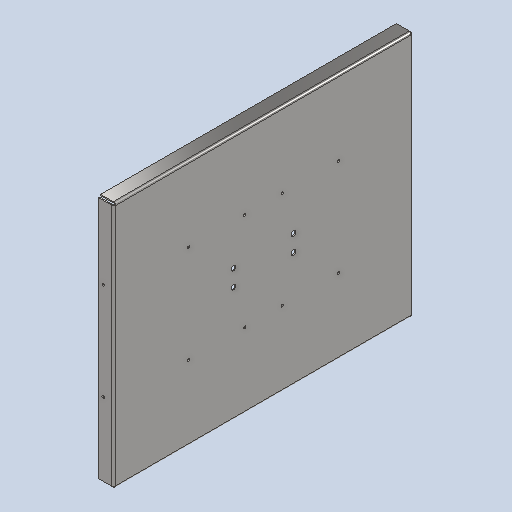
# Autodesk Inventor part: C_plate
Saved by Autodesk Inventor 2025.2 (Build 292293000, 293)
## iProperties
Created: 2025-04-08
Part Number: C_plate
Material: Stainless Steel
Document SubType Name: Sheet Metal
Designer: Caspe
Density: 8 g/cm^3
Sheet Metal Rule: Default_mm
Appearance: Semi-Polished
Flat Pattern Width: 36.4786 cm
Flat Pattern Length: 43.4786 cm
Flat Pattern Area: 1586.04 cm^2
Sheet Metal Width: 364,786 mm
Sheet Metal Length: 434,786 mm
Sheet Metal Area: 158603,718 mm^2
Mass: 1883.49 g
Surface Area: 3166.42 cm^2
Volume: 235.436 cm^3
Author: Caspe
Autodesk Inventor part; units mm, degrees
note: some values were not read from the file. Chosen so that the rebuilt part matches the saved one: corner form of "Plate2".
ref_plane "YZ Plane" through (0, 0, 0) normal (1, 0, 0) x (0, 1, 0)
ref_plane "XZ Plane" through (0, 0, 0) normal (0, 1, 0) x (-1, 0, 0)
ref_plane "XY Plane" through (0, 0, 0) normal (0, 0, 1) x (1, 0, 0)
sketch "Sketch1" plane through (0, 0, 0) normal (1, 0, 0) x (0, 1, 0)
  line L0 (165, 200) -> (-165, 200)
  line L1 (-165, 200) -> (-165, -200)
  line L2 (-165, -200) -> (165, -200)
  line L3 (165, -200) -> (165, 200)
  line L4 (165, 200) -> (-165, -200) construction
  line L5 (-165, 200) -> (165, -200) construction
  point P0 (0, 0)
  dimension "d0" = 330
  dimension "d1" = 400
  measures "d0" distance of L2.end L1.end
  measures "d1" distance of L1.end L0.end
extrude "Plate1" add sketch "Sketch1" along normal blind 1.5
sketch "Sketch2" plane through (1.5, 165, 198.5) normal (0, 0, 1) x (1, 0, 0)
  line L0 (0, -330) -> (0, 0)
  line L1 (0, 0) -> (-20, 0)
  line L2 (-20, 0) -> (-20, -330)
  line L3 (-20, -330) -> (0, -330)
  constraints: 6 end point, 1 horizontal, 1 perpendicular, 1 vertical
edge flange "Flange1" height 20 angle 90 thickness 1.5 bend radius 1.5 thickness toward (0, 0, 1) relief tear relief width 1.5 relief depth 0.75 corner gap 1.5 corner form 2 edges at (0, 0, 200) (0, 165, 0) (0, 0, -200) (0, -165, 0) wall of the first edge with corners at (1.5, -165, 198.5) (1.5, 165, 198.5) (-18.5, 165, 198.5) (-18.5, -165, 198.5)
bend "Bend1"
corner "Corner1"
sketch "Sketch4" plane through (0, 0, 0) normal (-1, 0, 0) x (0, 0, 1)
  circle A0 centre (-31.5, 11) radius 3.3
  line L0 (0, 0) -> (-5.5711, 0)
  line L1 (0, 0) -> (-6.9523, 0)
  line L2 (0, 0) -> (0, 7.85)
  circle A1 centre (-31, -11) radius 3.3
  circle A2 centre (31.5, 11) radius 3.3
  circle A3 centre (31, -11) radius 3.3
  dimension "d21" = 6.6
  dimension "d22" = 31.5
  dimension "d23" = 11
  dimension "d26" = 31
  dimension "d27" = 11
  dimension "d28" = 6.6
  constraints: 6 end point, 4 centre point, 2 horizontal, 2 symmetric about line, 1 vertical, 2 other
  measures "d21" diameter of A0
  measures "d22" horizontal distance of L0.start A0.centre
  measures "d23" vertical distance of L0.start A0.centre
  measures "d26" distance from line of A1.centre L2
  measures "d27" distance from line of L0 A1.centre
  measures "d28" diameter of A1
cut "Cut2" [suppressed]
sketch "Sketch5" plane through (0, 0, 0) normal (-1, 0, 0) x (0, 0, 1)
  line L0 (0, 0) -> (-12.9701, 0)
  line L1 (0, 0) -> (0, 9.9832)
  circle A0 centre (-25, 65) radius 1.7
  circle A1 centre (-100, 65) radius 1.7
  circle A2 centre (25, 65) radius 1.7
  circle A3 centre (100, 65) radius 1.7
  circle A4 centre (-25, -65) radius 1.7
  circle A5 centre (-100, -65) radius 1.7
  circle A6 centre (100, -65) radius 1.7
  circle A7 centre (25, -65) radius 1.7
  dimension "d29" = 3.4
  dimension "d30" = 65
  dimension "d31" = 50
  dimension "d32" = 3.4
  dimension "d33" = 65
  dimension "d34" = 200
  constraints: 8 centre point, 6 symmetric about line, 4 end point, 1 horizontal, 1 vertical, 6 other
  measures "d29" diameter of A0
  measures "d30" distance from line of L0 A0.centre
  measures "d31" diameter of A0.centre L1
  measures "d32" diameter of A1
  measures "d33" distance from line of L0 A1.centre
  measures "d34" diameter of A1.centre L1
sketch "Sketch7" plane through (-18.5, 162.4393, -198.5) normal (0, 0, 1) x (1, 0, 0)
  line L0 (17, -324.4393) -> (17, -0.4393) projected
  line L1 (17, -162.4393) -> (0, -162.4393)
  line L2 (0, 0) -> (0, -324.8787) projected
  circle A0 centre (6, -97.4393) radius 1.7
  circle A1 centre (6, -227.4393) radius 1.7
  line L3 (18.5, -162.4393) -> (18.5, -152.4561) projected
  point P0 (18.5, -162.4393)
  dimension "d35" = 3.4
  dimension "d36" = 6
  dimension "d42" = 65
  constraints: 2 centre point, 2 end point, 2 midpoint, 1 symmetric about line, 1 other
  measures "d35" diameter of A0
  measures "d36" distance from line of L2 A0.centre
  measures "d42" distance from line of A0.centre L1
extrude "Cut3" cut sketch "Sketch7" along normal through all both and the other way through all
extrude "Cut4" cut sketch "Sketch5" against normal through all
sketch "Sketch8" plane through (0, 0, 0) normal (-1, 0, 0) x (0, 0, 1)
  line L0 (0, 0) -> (0, 2.2695)
  line L1 (0, 0) -> (-3.4702, 0)
  circle A0 centre (-40, 11) radius 3.3
  circle A1 centre (40, 11) radius 3.3
  circle A2 centre (-40, -11) radius 3.3
  circle A3 centre (40, -11) radius 3.3
  dimension "d43" = 6.6
  dimension "d44" = 40
  dimension "d45" = 11
  constraints: 4 centre point, 4 end point, 3 symmetric about line, 1 horizontal, 1 vertical, 3 other
  measures "d43" diameter of A0
  measures "d44" distance from line of L0 A0.centre
  measures "d45" distance from line of L1 A0.centre
extrude "Cut5" cut sketch "Sketch8" against normal blind 1.5
equation "\"d0\" = C_height"
equation "\"d1\" = C_length"
equation "\"d24\" = Thickness"
equation "\"d32\" = d29"
equation "\"d33\" = d30"
equation "\"d35\" = d29"
equation "\"d42\" = d30"
equation "\"d38\" = Thickness"
equation "\"d40\" = Thickness"
equation "\"d46\" = Thickness"
equation "\"d2\" = Thickness"
equation "\"d3\" = BendReliefWidth"
equation "\"d4\" = BendReliefDepth"
equation "\"d5\" = MinimumRemnant"
equation "\"d6\" = TransitionRadius"
equation "\"d7\" = C_width"
equation "\"d9\" = BendRadius"
equation "\"d10\" = CornerReliefSize"
equation "\"d11\" = GapSize"
equation "\"d12\" = JacobiRadiusSize"
equation "\"BendRadius\" = Thickness"
equation "\"BendReliefWidth\" = Thickness"
equation "\"BendReliefDepth\" = 0.5 * Thickness"
equation "\"CornerReliefSize\" = 4 * Thickness"
equation "\"MinimumRemnant\" = 2 * Thickness"
equation "\"TransitionRadius\" = BendRadius"
equation "\"JacobiRadiusSize\" = BendRadius"
equation "\"GapSize\" = Thickness"
equation "\"A_width\" = 46"
equation "\"A_joint_diameter\" = 16"
equation "\"A_joint_tolerance\" = 3"
equation "\"l___________\" = 0"
equation "\"l__________\" = 0"
equation "\"C_length\" = 400"
equation "\"C_height\" = 330"
equation "\"l_________\" = 0"
equation "\"rivet_diameter\" = 3.35"
equation "\"plate_thickness\" = 3"
equation "\"l________\" = 0"
equation "\"A_B_spacing\" = 2"
equation "\"L_Piston_Bottom\" = 21"
equation "\"L_Piston_Top\" = 25"
equation "\"thin_plate\" = 1.5"
equation "\"Thickness\" = 1.5"
equation "\"C_width\" = 20"
body "Solid1"
